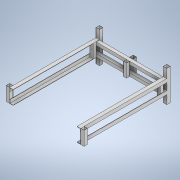
# Autodesk Inventor part: SoporteBobina
Saved by Autodesk Inventor 2020 (Build 240168000, 168)
## iProperties
Created: 2022-03-21
Part Number: SoporteBobina
Material: Genérico
Document SubType Name: Modeling
Designer: aarco
Density: 1 g/cm^3
Appearance: Valor por defecto
Mass: 5204.36 g
Surface Area: 21062.3 cm^2
Volume: 5204.36 cm^3
Author: aarco
Autodesk Inventor part; units mm, degrees
ref_plane "YZ Plane" through (0, 0, 0) normal (1, 0, 0) x (0, 1, 0)
ref_plane "XZ Plane" through (0, 0, 0) normal (0, 1, 0) x (-1, 0, 0)
ref_plane "XY Plane" through (0, 0, 0) normal (0, 0, 1) x (1, 0, 0)
sketch "Boceto1" plane through (0, 0, 0) normal (0, 0, 1) x (1, 0, 0)
  line L0 (0, 0) -> (-828.6689, 0) construction
  line L1 (0, 0) -> (821.843, 0) construction
  line L2 (-400, 150) -> (400, 150) construction
  line L3 (400, 150) -> (400, 0) construction
  line L4 (400, 0) -> (-400, 0) construction
  line L5 (-400, 0) -> (-400, 150) construction
  line L6 (0, 0) -> (0, 380.6015) construction
  line L7 (-404, 36) -> (-404, -4) construction
  line L8 (-404, -4) -> (-364, -4)
  line L9 (-364, -4) -> (-364, 0)
  line L10 (-364, 0) -> (-400, 0)
  line L11 (-400, 36) -> (-400, 0)
  line L12 (-404, 36) -> (-400, 36)
  line L13 (-404, -4) -> (-444, -4)
  line L14 (-444, -4) -> (-444, 36)
  line L15 (-444, 36) -> (-404, 36)
  line L16 (-404, 36) -> (-404, -4) construction
  line L17 (-442, 34) -> (-406, 34)
  line L18 (-406, 34) -> (-406, -2)
  line L19 (-406, -2) -> (-442, -2)
  line L20 (-442, -2) -> (-442, 34)
  line L21 (-424, 34) -> (-424, 36) construction
  line L22 (-442, 16) -> (-444, 16) construction
  line L23 (0, 0) -> (828.6689, 0) construction
  line L24 (0, 0) -> (-821.843, 0) construction
  line L25 (-400, 0) -> (400, 0) construction
  line L26 (404, 36) -> (404, -4) construction
  line L27 (404, -4) -> (364, -4)
  line L28 (364, -4) -> (364, 0)
  line L29 (364, 0) -> (400, 0)
  line L30 (400, 36) -> (400, 0)
  line L31 (404, 36) -> (400, 36)
  line L32 (404, -4) -> (444, -4)
  line L33 (444, -4) -> (444, 36)
  line L34 (444, 36) -> (404, 36)
  line L35 (404, 36) -> (404, -4) construction
  line L36 (442, 34) -> (406, 34)
  line L37 (406, 34) -> (406, -2)
  line L38 (406, -2) -> (442, -2)
  line L39 (442, -2) -> (442, 34)
  line L40 (424, 34) -> (424, 36) construction
  line L41 (442, 16) -> (444, 16) construction
  line L42 (400, 75) -> (-400, 75) construction
  line L43 (0, 150) -> (-828.6689, 150) construction
  line L44 (0, 150) -> (821.843, 150) construction
  line L45 (400, 150) -> (-400, 150) construction
  line L46 (0, 150) -> (0, -230.6015) construction
  line L47 (-404, 114) -> (-404, 154) construction
  line L48 (-404, 154) -> (-364, 154)
  line L49 (-364, 154) -> (-364, 150)
  line L50 (-364, 150) -> (-400, 150)
  line L51 (-400, 114) -> (-400, 150)
  line L52 (-404, 114) -> (-400, 114)
  line L53 (-404, 154) -> (-444, 154)
  line L54 (-444, 154) -> (-444, 114)
  line L55 (-444, 114) -> (-404, 114)
  line L56 (-404, 114) -> (-404, 154) construction
  line L57 (-442, 116) -> (-406, 116)
  line L58 (-406, 116) -> (-406, 152)
  line L59 (-406, 152) -> (-442, 152)
  line L60 (-442, 152) -> (-442, 116)
  line L61 (-424, 116) -> (-424, 114) construction
  line L62 (-442, 134) -> (-444, 134) construction
  line L63 (-400, 150) -> (400, 150) construction
  line L64 (364, 150) -> (400, 150)
  line L65 (364, 154) -> (364, 150)
  line L66 (404, 154) -> (364, 154)
  line L67 (0, 150) -> (828.6689, 150) construction
  line L68 (400, 114) -> (400, 150)
  line L69 (404, 114) -> (400, 114)
  line L70 (404, 114) -> (404, 154) construction
  line L71 (404, 114) -> (404, 154) construction
  line L72 (406, 116) -> (406, 152)
  line L73 (424, 116) -> (424, 114) construction
  line L74 (406, 152) -> (442, 152)
  line L75 (404, 154) -> (444, 154)
  line L76 (442, 152) -> (442, 116)
  line L77 (444, 154) -> (444, 114)
  line L78 (442, 134) -> (444, 134) construction
  line L79 (442, 116) -> (406, 116)
  line L80 (444, 114) -> (404, 114)
  line L81 (0, 150) -> (-821.843, 150) construction
  dimension "d0" = 800
  dimension "d1" = 150
  dimension "d3" = 4
  dimension "d5" = 40
  dimension "d7" = 40
  dimension "d8" = 2
  constraints: 164 end point, 60 symmetric about line, 12 perpendicular, 9 point on line, 6 midpoint, 6 parallel, 5 horizontal, 2 collinear, 2 vertical
  measures "d0" distance of L2.start L2.end
  measures "d1" distance of L4.end L2.start
  measures "d3" distance of L8.end L9.end
  measures "d5" distance between parallel lines of L8 L12
  measures "d7" distance of L13.end L14.end
  measures "d8" distance of L21.start L21.end
extrude "Extrusión1" add sketch "Boceto1" along normal blind 904
sketch "Boceto2" plane through (-400, 0, 0) normal (1, 0, 0) x (0, 0, -1)
  line L0 (0, 0) -> (0, 36) projected
  line L1 (0, 36) -> (-904, 36) projected
  line L2 (-904, 0) -> (-904, 36) projected
  line L3 (0, 0) -> (-904, 0) projected
  line L4 (0, 0) -> (0, 36) projected
  line L5 (0, 36) -> (-904, 36) projected
  line L6 (0, 0) -> (-36, 0)
  line L7 (-36, 0) -> (-36, 36)
  line L8 (-36, 36) -> (0, 36)
  line L9 (0, 36) -> (0, 0)
  line L10 (0, 114) -> (-904, 114) projected
  line L11 (0, 114) -> (-36, 114)
  line L12 (-36, 114) -> (-36, 150)
  line L13 (-36, 150) -> (0, 150)
  line L14 (0, 150) -> (0, 114)
  line L15 (0, 150) -> (-904, 150) projected
  constraints: 16 end point, 4 parallel, 4 perpendicular, 2 horizontal, 2 point on line
extrude "Extrusión2" add sketch "Boceto2" along normal up to next contours L3 L7 L1 L0 | L10 L12 L13 L14
sketch "Boceto10" plane through (0, 0, 904) normal (0, 0, 1) x (1, 0, 0)
  line L0 (-400, 114) -> (-400, 150) projected
  line L1 (-400, 150) -> (-364, 150) projected
  line L2 (-364, 150) -> (-364, 154) projected
  line L3 (-364, 154) -> (-444, 154) projected
  line L4 (-444, 154) -> (-444, 114) projected
  line L5 (-444, 114) -> (-400, 114) projected
  line L6 (-442, 152) -> (-406, 152) projected
  line L7 (-406, 152) -> (-406, 116) projected
  line L8 (-406, 116) -> (-442, 116) projected
  line L9 (-442, 116) -> (-442, 152) projected
  line L10 (-400, 36) -> (-444, 36) projected
  line L11 (-444, 36) -> (-444, -4) projected
  line L12 (-444, -4) -> (-364, -4) projected
  line L13 (-364, -4) -> (-364, 0) projected
  line L14 (-364, 0) -> (-400, 0) projected
  line L15 (-400, 0) -> (-400, 36) projected
  line L16 (-442, -2) -> (-442, 34) projected
  line L17 (-442, 34) -> (-406, 34) projected
  line L18 (-406, 34) -> (-406, -2) projected
  line L19 (-406, -2) -> (-442, -2) projected
  line L20 (400, 114) -> (444, 114) projected
  line L21 (444, 114) -> (444, 154) projected
  line L22 (444, 154) -> (364, 154) projected
  line L23 (364, 154) -> (364, 150) projected
  line L24 (364, 150) -> (400, 150) projected
  line L25 (400, 150) -> (400, 114) projected
  line L26 (442, 152) -> (442, 116) projected
  line L27 (442, 116) -> (406, 116) projected
  line L28 (406, 116) -> (406, 152) projected
  line L29 (406, 152) -> (442, 152) projected
  line L30 (400, 36) -> (400, 0) projected
  line L31 (400, 0) -> (364, 0) projected
  line L32 (364, 0) -> (364, -4) projected
  line L33 (364, -4) -> (444, -4) projected
  line L34 (444, -4) -> (444, 36) projected
  line L35 (444, 36) -> (400, 36) projected
  line L36 (442, 34) -> (442, -2) projected
  line L37 (442, -2) -> (406, -2) projected
  line L38 (406, -2) -> (406, 34) projected
  line L39 (406, 34) -> (442, 34) projected
  line L40 (-364, 154) -> (-444, 154) projected
  line L41 (-404, 154) -> (-404, -4)
  line L42 (-444, -4) -> (-364, -4) projected
  line L43 (404, -4) -> (404, 154)
  line L44 (444, 154) -> (364, 154) projected
  point P0 (0, 0)
  point P1 (404, 114)
  point P2 (404, 36)
  point P3 (-404, 114)
  point P4 (-404, -4)
  point P5 (-404, 36)
  dimension "d36" = 2
  dimension "d37" = 2
  constraints: 4 end point, 3 midpoint, 1 perpendicular, 1 vertical
  measures "d36" distance between parallel lines of L18 L41
  measures "d37" distance between parallel lines of L43 L28
extrude "Extrusión5" add sketch "Boceto10" along normal blind 40 contours L5 L4 L3 L41 | L41 L12 L11 L10 | L43 L22 L21 L20 | L35 L34 L33 L43
sketch "Boceto15" plane through (-444, -4, 0) normal (0, -1, 0) x (1, 0, 0)
  line L0 (0, 0) -> (0, 944) projected
  line L1 (0, 0) -> (80, 0)
  line L2 (808, 0) -> (808, -40)
  line L3 (808, -40) -> (848, -40)
  line L4 (810, -2) -> (846, -2)
  line L5 (846, -2) -> (846, -38)
  line L6 (846, -38) -> (810, -38)
  line L7 (810, -38) -> (810, -2)
  line L8 (808, -20) -> (810, -20) construction
  line L9 (828, -38) -> (828, -40) construction
  line L10 (424, 0) -> (464, 0)
  line L11 (464, 0) -> (464, -40)
  line L12 (464, -40) -> (424, -40)
  line L13 (424, -40) -> (424, 0)
  line L14 (426, -2) -> (462, -2)
  line L15 (462, -2) -> (462, -38)
  line L16 (462, -38) -> (426, -38)
  line L17 (426, -38) -> (426, -2)
  line L18 (424, -20) -> (426, -20) construction
  line L19 (444, -38) -> (444, -40) construction
  line L20 (80, 0) -> (0, 0) projected
  line L21 (0, 0) -> (80, 0) projected
  line L22 (80, 0) -> (40, 0)
  line L23 (40, 0) -> (40, -40)
  line L24 (40, -40) -> (80, -40)
  line L25 (80, -40) -> (80, 0)
  line L26 (42, -2) -> (78, -2)
  line L27 (78, -2) -> (78, -38)
  line L28 (78, -38) -> (42, -38)
  line L29 (42, -38) -> (42, -2)
  line L30 (42, -20) -> (40, -20)
  line L31 (60, -38) -> (60, -40)
  line L32 (848, -40) -> (848, 0)
  line L33 (80, 0) -> (808, 0) projected
  line L34 (888, 0) -> (808, 0) projected
  point P0 (444, 0)
  point P1 (444, 0)
  dimension "d48" = 2
  dimension "d51" = 2
  dimension "d52" = 40
  dimension "d82" = 2
  dimension "d83" = 40
  dimension "d84" = 40
  constraints: 60 end point, 18 perpendicular, 14 midpoint, 10 parallel, 6 horizontal, 1 coincident, 1 vertical
  measures "d48" distance between parallel lines of L2 L7
  measures "d51" distance of L18.start L18.end
  measures "d52" distance of L12.end L10.start
  measures "d82" distance of L30.start L30.end
  measures "d83" distance of L22.end L23.end
  measures "d84" distance of L32.end L3.end
extrude "Extrusión8" add sketch "Boceto15" against normal up to surface (158 mm away) contours L1 L25 L24 L31 L28 L27 L26 L29 L30 L23 | L30 L29 L28 L31 L24 L23 | L34 L32 L3 L2 | L10 L11 L12 L13
sketch "Boceto16" plane through (-364, -4, 0) normal (0, -1, 0) x (1, 0, 0)
  line L0 (-80, 0) -> (-40, 0) projected
  line L1 (-40, 904) -> (0, 904) projected
  line L2 (-40, 904) -> (-40, 944) projected
  line L3 (-80, 944) -> (-40, 944) projected
  line L4 (-80, 0) -> (-80, 944) projected
  line L5 (768, 0) -> (808, 0) projected
  line L6 (808, 0) -> (808, 944) projected
  line L7 (768, 944) -> (808, 944) projected
  line L8 (768, 904) -> (768, 944) projected
  line L9 (728, 904) -> (768, 904) projected
  line L10 (0, -40) -> (0, 904) projected
  line L11 (-40, 0) -> (-40, -40) projected
  line L12 (-38, -38) -> (-38, -2) projected
  line L13 (-38, -2) -> (-2, -2) projected
  line L14 (-2, -2) -> (-2, -38) projected
  line L15 (-2, -38) -> (-38, -38) projected
  line L16 (-40, -40) -> (0, -40) projected
  line L17 (-40, 0) -> (0, 0)
  line L18 (728, -40) -> (728, 904) projected
  line L19 (728, -40) -> (768, -40) projected
  line L20 (768, -40) -> (768, 0) projected
  line L21 (808, 0) -> (768, 0) projected
  line L22 (728, 0) -> (768, 0) projected
  line L23 (768, 0) -> (728, 0)
  line L24 (730, -2) -> (766, -2) projected
  line L25 (730, -38) -> (730, -2) projected
  line L26 (766, -2) -> (766, -38) projected
  line L27 (766, -38) -> (730, -38) projected
  point P0 (364, 0)
  constraints: 4 end point, 2 horizontal
extrude "Extrusión9" add sketch "Boceto16" along normal blind 100 contours L17 L10 L16 L11 | L20 L19 L18 L22
sketch "Boceto18" plane through (-400, 150, 904) normal (0, -1, 0) x (1, 0, 0)
  line L0 (0, -868) -> (0, 0) projected
  line L1 (36, -868) -> (36, 0) projected
  line L2 (0, -868) -> (36, -868)
  line L3 (36, -868) -> (36, -832)
  line L4 (36, -832) -> (0, -832)
  line L5 (0, -832) -> (0, -868)
  line L6 (764, -868) -> (800, -868) projected
  line L7 (764, -868) -> (764, 0) projected
  line L8 (800, -868) -> (764, -868)
  line L9 (764, -868) -> (764, -832)
  line L10 (764, -832) -> (800, -832)
  line L11 (800, -832) -> (800, -868)
  line L12 (36, -868) -> (764, -868) projected
  line L13 (382, -868) -> (418, -868)
  line L14 (418, -868) -> (418, -832)
  line L15 (418, -832) -> (382, -832)
  line L16 (382, -832) -> (382, -868)
  line L17 (384, -834) -> (416, -834)
  line L18 (416, -834) -> (416, -866)
  line L19 (416, -866) -> (384, -866)
  line L20 (384, -866) -> (384, -834)
  line L21 (400, -832) -> (400, -834) construction
  line L22 (384, -850) -> (382, -850) construction
  point P0 (400, -904)
  point P1 (400, -868)
  point P2 (0, -832)
  dimension "d55" = 2
  constraints: 36 end point, 9 perpendicular, 8 parallel, 6 midpoint, 5 point on line, 4 horizontal
  measures "d55" distance of L21.start L21.end
extrude "Extrusión10" add sketch "Boceto18" along normal up to surface (150 mm away)
sketch "Boceto19" plane through (364, 154, 904) normal (0, 1, 0) x (1, 0, 0)
  line L0 (80, 904) -> (40, 904) projected
  line L1 (0, 944) -> (0, 0) projected
  line L2 (40, 0) -> (0, 0) projected
  line L3 (40, 0) -> (40, -40) projected
  line L4 (80, -40) -> (40, -40) projected
  line L5 (80, 904) -> (80, -40) projected
  line L6 (-764, 868) -> (-728, 868) projected
  line L7 (-768, 904) -> (-808, 904) projected
  line L8 (-728, 944) -> (-728, 0) projected
  line L9 (-768, -40) -> (-808, -40) projected
  line L10 (-768, 0) -> (-768, -40) projected
  line L11 (-728, 0) -> (-768, 0) projected
  line L12 (-808, 904) -> (-808, -40) projected
  line L13 (-768, 944) -> (-728, 944) projected
  line L14 (-730, 942) -> (-766, 942) projected
  line L15 (-730, 906) -> (-730, 942) projected
  line L16 (-766, 906) -> (-730, 906) projected
  line L17 (-766, 942) -> (-766, 906) projected
  line L18 (-768, 904) -> (-768, 944) projected
  line L19 (-768, 904) -> (-808, 904) projected
  line L20 (-768, 904) -> (-728, 904) projected
  line L21 (-768, 904) -> (-728, 904)
  line L22 (38, 906) -> (38, 942) projected
  line L23 (2, 906) -> (38, 906) projected
  line L24 (2, 942) -> (2, 906) projected
  line L25 (38, 942) -> (2, 942) projected
  line L26 (0, 944) -> (0, 0) projected
  line L27 (40, 944) -> (40, 904) projected
  line L28 (0, 944) -> (40, 944) projected
  line L29 (40, 944) -> (40, 904) projected
  line L30 (0, 944) -> (40, 944) projected
  line L31 (80, 904) -> (40, 904) projected
  line L32 (40, 0) -> (0, 0) projected
  line L33 (40, 0) -> (40, -40) projected
  line L34 (80, -40) -> (40, -40) projected
  line L35 (80, 904) -> (80, -40) projected
  line L36 (-344, 904) -> (0, 904) projected
  line L37 (40, 904) -> (0, 904)
  point P0 (-364, 904)
  constraints: 4 end point, 1 collinear, 1 horizontal, 1 point on line
extrude "Extrusión11" add sketch "Boceto19" along normal blind 100 contours L37 L1 L28 L27 | L18 L13 L8 L20
sketch "Boceto22" plane through (364, 154, 904) normal (0, 1, 0) x (1, 0, 0)
  line L0 (40, -40) -> (80, -40) projected
  line L1 (80, -40) -> (40, -40)
  line L2 (40, -40) -> (40, -80)
  line L3 (40, -80) -> (80, -80)
  line L4 (80, -80) -> (80, -40)
  line L5 (-808, -40) -> (-768, -40)
  line L6 (-768, -40) -> (-768, -80)
  line L7 (-768, -80) -> (-808, -80)
  line L8 (-808, -80) -> (-808, -40)
  line L9 (78, -78) -> (42, -78)
  line L10 (42, -78) -> (42, -42)
  line L11 (42, -42) -> (78, -42)
  line L12 (78, -42) -> (78, -78)
  line L13 (60, -78) -> (60, -80) construction
  line L14 (78, -60) -> (80, -60) construction
  line L15 (-770, -78) -> (-806, -78)
  line L16 (-806, -78) -> (-806, -42)
  line L17 (-806, -42) -> (-770, -42)
  line L18 (-770, -42) -> (-770, -78)
  line L19 (-788, -78) -> (-788, -80) construction
  line L20 (-770, -60) -> (-768, -60) construction
  point P0 (-364, 904)
  dimension "d70" = 40
  dimension "d71" = 2
  dimension "d72" = 2
  constraints: 40 end point, 12 perpendicular, 8 midpoint, 8 parallel, 4 horizontal, 1 coincident
  measures "d70" distance of L2.end L3.end
  measures "d71" distance between parallel lines of L8 L16
  measures "d72" distance between parallel lines of L4 L12
extrude "Extrusión13" add sketch "Boceto22" against normal up to surface (158 mm away)
sketch "Boceto23" plane through (0, 0, 904) normal (0, 0, 1) x (1, 0, 0)
  line L0 (-404, 154) -> (-404, 114) projected
  line L1 (-404, 114) -> (-400, 114) projected
  line L2 (-400, 114) -> (-400, 150) projected
  line L3 (-400, 150) -> (-364, 150) projected
  line L4 (-364, 150) -> (-364, 154) projected
  line L5 (-404, 36) -> (-404, -4) projected
  line L6 (-364, -4) -> (-364, 0) projected
  line L7 (-364, 0) -> (-400, 0) projected
  line L8 (-400, 0) -> (-400, 36) projected
  line L9 (-400, 36) -> (-404, 36) projected
  line L10 (404, 114) -> (404, 154) projected
  line L11 (364, 154) -> (364, 150) projected
  line L12 (364, 150) -> (400, 150) projected
  line L13 (400, 150) -> (400, 114) projected
  line L14 (400, 114) -> (404, 114) projected
  line L15 (404, -4) -> (404, 36) projected
  line L16 (404, 36) -> (400, 36) projected
  line L17 (400, 36) -> (400, 0) projected
  line L18 (400, 0) -> (364, 0) projected
  line L19 (364, 0) -> (364, -4) projected
  line L20 (364, -4) -> (404, -4) projected
  line L21 (-364, 154) -> (-404, 154) projected
  line L22 (-404, -4) -> (-364, -4) projected
  line L23 (404, 154) -> (364, 154) projected
  point P0 (0, 0)
extrude "Extrusión14" add sketch "Boceto23" along normal up to surface (80 mm away)
sketch "Boceto24" plane through (-444, -104, 0) normal (-1, 0, 0) x (0, 0, -1)
  line L0 (0, -140) -> (-944, -140) projected
  line L1 (0, -218) -> (-944, -218) projected
  line L2 (-944, -218) -> (-944, -140) projected
  line L3 (-984, -258) -> (-984, -100) projected
  line L4 (0, -258) -> (-984, -258) projected
  line L5 (-944, -218) -> (0, -218)
  line L6 (-944, -218) -> (-944, -140) projected
  line L7 (-944, -140) -> (0, -140)
  line L8 (0, -258) -> (0, -218) projected
  line L9 (-944, -218) -> (-944, -140) projected
  line L10 (-944, -140) -> (-944, -100)
  line L11 (-944, -218) -> (-944, -258)
  line L12 (0, -140) -> (0, -100) projected
  line L13 (0, -100) -> (-984, -100) projected
  point P0 (0, -104)
  point P1 (0, 100)
  point P2 (0, 258)
  point P3 (-775.1193, -140)
  point P4 (0, -218)
  point P5 (-944, -100)
  point P6 (0, -140)
  constraints: 8 end point, 2 point on line, 1 horizontal
extrude "Extrusión15" cut sketch "Boceto24" against normal blind 40 contours L0 L10 L13 L12 | L1 L8 L4 L11
sketch "Boceto25" plane through (444, -104, 0) normal (1, 0, 0) x (0, 0, -1)
  line L0 (-944, 218) -> (-944, 140) projected
  line L1 (0, 258) -> (-984, 258) projected
  line L2 (-944, 258) -> (0, 258)
  line L3 (0, 258) -> (0, 100)
  line L4 (0, 100) -> (-944, 100)
  line L5 (-944, 100) -> (-944, 258)
  point P0 (0, 104)
  point P1 (-944, 218)
  constraints: 8 end point, 2 parallel, 2 point on line, 1 horizontal, 1 perpendicular
extrude "Extrusión16" cut sketch "Boceto25" against normal blind 40
